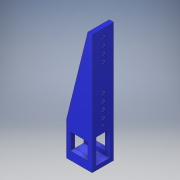
# Autodesk Inventor part: TopRearLeg
Saved by Autodesk Inventor 2019 (Build 230136000, 136)
## iProperties
Created: 2019-03-31
Part Number: TopRearLeg
Material: Generic
Document SubType Name: Modeling
Designer: cnam
Density: 1 g/cm^3
Appearance: Default
Author: cnam
Autodesk Inventor part; units mm, degrees
ref_plane "YZ Plane" through (0, 0, 0) normal (1, 0, 0) x (0, 1, 0)
ref_plane "XZ Plane" through (0, 0, 0) normal (0, 1, 0) x (-1, 0, 0)
ref_plane "XY Plane" through (0, 0, 0) normal (0, 0, 1) x (1, 0, 0)
sketch "Sketch1" plane through (0, 0, 0) normal (1, 0, 0) x (0, 1, 0)
  line L0 (47.75, -10) -> (-47.75, -10)
  line L1 (-47.75, -10) -> (-47.75, 10)
  line L2 (-47.75, 10) -> (47.75, 10)
  line L3 (47.75, 10) -> (47.75, -10)
  line L4 (47.75, -10) -> (-47.75, 10) construction
  line L5 (-47.75, -10) -> (47.75, 10) construction
  circle A0 centre (40.75, 0) radius 2
  circle A1 centre (-4.25, 0) radius 2
  line L6 (18.25, 25.1028) -> (18.25, -34.7635) construction
  line L7 (-1.75, 23.8417) -> (-1.75, -36.7999) construction
  circle A2 centre (20.75, 0) radius 2
  circle A3 centre (-24.25, 0) radius 2
  line L8 (-41.75, 23.8417) -> (-41.75, -30.9921) construction
  circle A4 centre (34.0833, 0) radius 2
  circle A5 centre (27.4167, 0) radius 2
  circle A6 centre (-10.9167, 0) radius 2
  circle A7 centre (-17.5833, 0) radius 2
  point P0 (0, 0)
  dimension "d1" = 20
  dimension "d4" = 4
  dimension "d5" = 7
  dimension "d6" = 45
  dimension "d7" = 22.5
  dimension "d8" = 20
  dimension "d9" = 22.5
  dimension "d10" = 22.5
  dimension "d11" = 60
  dimension "d18" = 6.6667
  dimension "d25" = 6.6667
  dimension "d30" = 6
  constraints: 18 end point, 8 centre point, 3 equal radius, 3 horizontal, 3 vertical, 2 midpoint, 2 parallel, 1 perpendicular, 8 other
  measures "d1" distance of L2.end L0.start
  measures "d4" diameter of A0
  measures "d5" distance from line of L3 A0.centre
  measures "d6" distance of A1.centre A0.centre
  measures "d7" distance from line of L6 A0.centre
  measures "d8" distance between parallel lines of L6 L7
  measures "d9" distance from line of L7 A2.centre
  measures "d10" distance from line of L7 A3.centre
  measures "d11" distance between parallel lines of L8 L6
  measures "d18" distance of A0.centre A4.centre
  measures "d25" distance of A1.centre A6.centre
  measures "d30" distance between parallel lines of L8 L1
extrude "Extrusion1" add sketch "Sketch1" along normal blind 4
sketch "Sketch2" plane through (0, 0, 0) normal (1, 0, 0) x (0, 1, 0)
  line L0 (-41.75, 22.3574) -> (-41.75, -36.9148) construction
  circle A0 centre (-17.5833, 0) radius 2 projected
  circle A1 centre (-10.9167, 0) radius 2 projected
  circle A2 centre (27.4167, 0) radius 2 projected
  circle A3 centre (34.0833, 0) radius 2 projected
  circle A4 centre (-24.25, 0) radius 2 projected
  circle A5 centre (20.75, 0) radius 2 projected
  circle A6 centre (-4.25, 0) radius 2 projected
  circle A7 centre (40.75, 0) radius 2 projected
  line L1 (-47.75, -10) -> (47.75, -10) projected
  line L2 (47.75, -10) -> (47.75, 10) projected
  line L3 (47.75, 10) -> (-47.75, 10) projected
  line L4 (-47.75, 10) -> (-47.75, -10) projected
  line L5 (47.75, 0) -> (-47.75, 0) construction
  line L6 (-47.75, -10) -> (-47.75, 10) projected
  line L7 (-59.75, -6.125) -> (-36.75, -6.125)
  line L8 (-36.75, -6.125) -> (-36.75, 6.125)
  line L9 (-36.75, 6.125) -> (-59.75, 6.125)
  line L10 (-59.75, 6.125) -> (-59.75, -6.125)
  line L11 (-59.75, -6.125) -> (-36.75, 6.125) construction
  line L12 (-36.75, -6.125) -> (-59.75, 6.125) construction
  line L13 (-47.75, -10) -> (-63.625, -10)
  line L14 (-63.625, -10) -> (-63.625, 10)
  line L15 (-63.625, 10) -> (-47.75, 10)
  line L16 (-47.75, 10) -> (-47.75, -10)
  line L17 (-32.875, -10) -> (-32.875, 10)
  point P0 (0, 0)
  point P1 (-48.25, 0)
  dimension "d33" = 6
  dimension "d34" = 12.25
  dimension "d35" = 23
  dimension "d36" = 5
  dimension "d37" = 3.875
  dimension "d38" = 3.875
  dimension "d39" = 3.875
  constraints: 26 end point, 4 midpoint, 4 parallel, 3 perpendicular, 3 point on line, 2 horizontal, 1 vertical
  measures "d33" distance between parallel lines of L4 L0
  measures "d34" distance of L7.end L8.end
  measures "d35" distance of L7.start L7.end
  measures "d36" distance between parallel lines of L0 L8
  measures "d37" distance between parallel lines of L15 L9
  measures "d38" distance between parallel lines of L14 L10
  measures "d39" distance between parallel lines of L8 L17
extrude "Extrusion2" cut sketch "Sketch2" along normal blind 20 contours L7 L10 L9 L4 | L4 L9 L8 L7
sketch "Sketch3" plane through (0, 0, 0) normal (-1, 0, 0) x (0, 0, 1)
  line L0 (-10, -47.75) -> (-6.125, -47.75) projected
  line L1 (-10, -47.75) -> (-6.125, -47.75)
  line L2 (6.125, -47.75) -> (10, -47.75) projected
  line L3 (10, -47.75) -> (6.125, -47.75)
  line L4 (6.125, -36.75) -> (6.125, -47.75) projected
  line L5 (6.125, -47.75) -> (10, -47.75) projected
  line L6 (10, -47.75) -> (10, 47.75) projected
  line L7 (10, 47.75) -> (-10, 47.75) projected
  line L8 (-10, 47.75) -> (-10, -47.75) projected
  line L9 (-10, -47.75) -> (-6.125, -47.75) projected
  line L10 (-6.125, -47.75) -> (-6.125, -36.75) projected
  line L11 (-6.125, -36.75) -> (6.125, -36.75) projected
  circle A0 centre (0, -17.5833) radius 2 projected
  circle A1 centre (0, -10.9167) radius 2 projected
  circle A2 centre (0, 27.4167) radius 2 projected
  circle A3 centre (0, 34.0833) radius 2 projected
  circle A4 centre (0, -24.25) radius 2 projected
  circle A5 centre (0, 20.75) radius 2 projected
  circle A6 centre (0, -4.25) radius 2 projected
  circle A7 centre (0, 40.75) radius 2 projected
  line L12 (-6.125, -36.75) -> (6.125, -36.75)
  line L13 (6.125, -36.75) -> (6.125, -59.75)
  line L14 (6.125, -59.75) -> (-6.125, -59.75)
  line L15 (-6.125, -59.75) -> (-6.125, -36.75)
  line L16 (-10, 47.75) -> (-10, -47.75) projected
  line L17 (-10, -32.875) -> (10, -32.875)
  line L18 (10, -32.875) -> (10, -63.625)
  line L19 (10, -63.625) -> (-10, -63.625)
  line L20 (-10, -63.625) -> (-10, -32.875)
  point P0 (0, 0)
  dimension "d44" = 23
  dimension "d45" = 3.875
  dimension "d46" = 3.875
  dimension "d47" = 3.875
  constraints: 20 end point, 5 equal length, 3 horizontal, 2 perpendicular, 1 point on line
  measures "d44" distance of L12.end L13.end
  measures "d45" distance between parallel lines of L12 L17
  measures "d46" distance between parallel lines of L19 L14
  measures "d47" distance between parallel lines of L18 L13
extrude "Extrusion4" add sketch "Sketch3" along normal blind 20 contours L8 L17 L6 L2 L4 L11 L10 L0 | L0 L15 L14 L13 L2 L18 L19 L20
sketch "Sketch5" plane through (0, 0, 0) normal (1, 0, 0) x (0, 0, -1)
  line L0 (-6.125, -47.75) -> (-10, -47.75) projected
  line L1 (-10, -63.625) -> (-10, -47.75) projected
  line L2 (10, -63.625) -> (-10, -63.625) projected
  line L3 (10, -47.75) -> (10, -63.625) projected
  line L4 (10, -47.75) -> (6.125, -47.75) projected
  line L5 (6.125, -47.75) -> (6.125, -59.75) projected
  line L6 (6.125, -59.75) -> (-6.125, -59.75) projected
  line L7 (-6.125, -59.75) -> (-6.125, -47.75) projected
  point P0 (0, 0)
extrude "Extrusion5" add sketch "Sketch5" along normal blind 4
sketch "Sketch6" plane through (0, 0, 0) normal (-1, 0, 0) x (0, 0, 1)
  line L0 (-10, -32.875) -> (10, -32.875) projected
  line L1 (10, -32.875) -> (10, 47.75) projected
  line L2 (10, 47.75) -> (-10, 47.75) projected
  line L3 (-10, 47.75) -> (-10, -32.875) projected
  circle A0 centre (0, -17.5833) radius 2 projected
  circle A1 centre (0, -10.9167) radius 2 projected
  circle A2 centre (0, 27.4167) radius 2 projected
  circle A3 centre (0, 34.0833) radius 2 projected
  circle A4 centre (0, -24.25) radius 2 projected
  circle A5 centre (0, 20.75) radius 2 projected
  circle A6 centre (0, -4.25) radius 2 projected
  circle A7 centre (0, 40.75) radius 2 projected
  circle A8 centre (0, -30.375) radius 0.875
  point P0 (0, 0)
  dimension "d52" = 2.5
  dimension "d53" = 1.75
  constraints: 1 centre point
  measures "d52" distance from line of L0 A8.centre
  measures "d53" diameter of A8
extrude "Extrusion6" cut sketch "Sketch6" against normal blind 4 contours A8
sketch "Sketch7" plane through (0, 47.75, 10) normal (0, 0, 1) x (1, 0, 0)
  line L0 (4, 0) -> (4, -111.375) projected
  line L1 (0, 0) -> (4, 0) projected
  line L2 (0, -80.625) -> (0, 0) projected
  line L3 (0, -80.625) -> (-20, -80.625) projected
  line L4 (-20, -111.375) -> (-20, -80.625) projected
  line L5 (4, -111.375) -> (-20, -111.375) projected
  line L6 (4, -84.5) -> (4, -107.5) projected
  line L7 (-20, -84.5) -> (4, -84.5) projected
  line L8 (-20, -107.5) -> (-20, -84.5) projected
  line L9 (4, -107.5) -> (-20, -107.5) projected
  line L10 (-16.125, -88.375) -> (0.125, -88.375)
  line L11 (0.125, -88.375) -> (0.125, -103.625)
  line L12 (0.125, -103.625) -> (-16.125, -103.625)
  line L13 (-16.125, -103.625) -> (-16.125, -88.375)
  point P0 (0, -47.75)
  dimension "d56" = 3.875
  dimension "d57" = 3.875
  dimension "d58" = 3.875
  dimension "d59" = 3.875
  constraints: 8 end point, 2 parallel, 1 horizontal, 1 perpendicular
  measures "d56" distance between parallel lines of L13 L4
  measures "d57" distance between parallel lines of L0 L11
  measures "d58" distance between parallel lines of L7 L10
  measures "d59" distance between parallel lines of L9 L12
extrude "Extrusion7" cut sketch "Sketch7" against normal blind 20 contours L10 L11 L12 L13
sketch "Sketch8" plane through (4, 47.75, -10) normal (0, 0, -1) x (-1, 0, 0)
  line L0 (24, -84.5) -> (0, -84.5) projected
  line L1 (20.125, -88.375) -> (20.125, -103.625) projected
  line L2 (20.125, -103.625) -> (3.875, -103.625) projected
  line L3 (3.875, -103.625) -> (3.875, -88.375) projected
  line L4 (3.875, -88.375) -> (20.125, -88.375) projected
  line L5 (4, 0) -> (4, -80.625) projected
  line L6 (4, 0) -> (0, 0) projected
  line L7 (0, -111.375) -> (0, 0) projected
  line L8 (0, -111.375) -> (24, -111.375) projected
  line L9 (24, -80.625) -> (24, -111.375) projected
  line L10 (4, -80.625) -> (24, -80.625) projected
  line L11 (4, -80.625) -> (4, 0) projected
  line L12 (4, 0) -> (4, -80.625) projected
  line L13 (24, -80.625) -> (4, 0)
  point P0 (4, -47.75)
  constraints: 2 end point
extrude "Extrusion8" add sketch "Sketch8" against normal blind 3 contours L10 L5 L13
mirror "Mirror2" about plane through (0, 0, 0) normal (0, 0, 1) of "Extrusion8"
sketch "Sketch9" plane through (4, 0, 0) normal (1, 0, 0) x (0, 0, -1)
  circle A0 centre (0, -30.375) radius 0.875 projected
  line L0 (10, -63.625) -> (10, 47.75) projected
  line L1 (10, 47.75) -> (-10, 47.75) projected
  line L2 (-10, 47.75) -> (-10, -63.625) projected
  line L3 (-10, -63.625) -> (10, -63.625) projected
  line L4 (6.125, -36.75) -> (6.125, -59.75) projected
  line L5 (6.125, -59.75) -> (-6.125, -59.75) projected
  line L6 (-6.125, -59.75) -> (-6.125, -36.75) projected
  line L7 (-6.125, -36.75) -> (6.125, -36.75) projected
  circle A1 centre (0, 40.75) radius 2 projected
  circle A2 centre (0, -4.25) radius 2 projected
  circle A3 centre (0, 20.75) radius 2 projected
  circle A4 centre (0, -24.25) radius 2 projected
  circle A5 centre (0, 34.0833) radius 2 projected
  circle A6 centre (0, 27.4167) radius 2 projected
  circle A7 centre (0, -10.9167) radius 2 projected
  circle A8 centre (0, -17.5833) radius 2 projected
  point P0 (0, 0)
body "Solid1"
